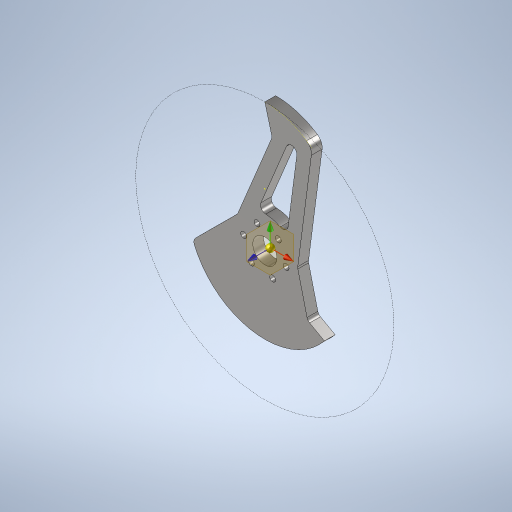
# Autodesk Inventor part: Blade
Saved by Autodesk Inventor 2023.4 (Build 274418000, 418)
## iProperties
Created: 2023-11-12
Part Number: Blade
Material: Steel, Alloy
Document SubType Name: Modeling
Designer: Nathan Cai
Density: 7.73 g/cm^3
Appearance: Semi-Polished
Mass: 199.265 g
Surface Area: 116.36 cm^2
Volume: 25.7782 cm^3
Author: Nathan Cai
Autodesk Inventor part; units mm, degrees
ref_plane "YZ Plane" through (0, 0, 0) normal (1, 0, 0) x (0, 1, 0)
ref_plane "XZ Plane" through (0, 0, 0) normal (0, 1, 0) x (-1, 0, 0)
ref_plane "XY Plane" through (0, 0, 0) normal (0, 0, 1) x (1, 0, 0)
sketch "Sketch1" plane through (0, 0, 0) normal (0, 0, 1) x (1, 0, 0)
  circle A0 centre (0, 0) radius 76.2 construction
  circle A1 centre (0, 0) radius 7.1437
  circle A2 centre (0, 0) radius 12.7 construction
  circle A3 centre (0, 0) radius 19.05
  line L0 (0, 76.2) -> (0, 0) construction
  line L1 (0, 76.2) -> (4.2947, 60.1719)
  line L2 (4.2947, 60.1719) -> (-17.6011, 7.2873)
  circle A4 centre (0, 0) radius 60.325 construction
  arc A5 (27.9352, 66.3249) -> (0, 76.2) centre (0, 31.75) ccw
  line L3 (27.9352, 66.3249) -> (18.8874, -2.4836)
  circle A6 centre (0, 0) radius 45.2437 construction
  line L4 (35.161, -28.4728) -> (0, 0) construction
  line L5 (35.161, -28.4728) -> (25.2413, -22.9743)
  line L6 (25.2413, -22.9743) -> (18.5029, 4.5327)
  circle A7 centre (0, 0) radius 34.1313 construction
  arc A8 (-42.5152, -15.4743) -> (35.161, -28.4728) centre (0, 0) ccw
  line L7 (-42.5152, -15.4743) -> (-13.4471, 13.4936)
  line L8 (-42.5152, -15.4743) -> (0, 0) construction
  line L9 (-4.3483, 18.5471) -> (12.7964, 59.9565)
  line L10 (13.0349, 13.8922) -> (18.8778, 58.328)
  arc A9 (18.8778, 58.328) -> (12.7964, 59.9565) centre (15.7299, 58.7419) ccw
  line L11 (-10.5541, 7.064) -> (0, 0) construction
  line L12 (0, 0) -> (-4.5937, 11.8401) construction
  circle A10 centre (-4.5937, 11.8401) radius 1.7526
  circle A11 centre (-12.5507, 1.9418) radius 1.7526
  circle A12 centre (-7.957, -9.8983) radius 1.7526
  circle A13 centre (4.5937, -11.8401) radius 1.7526
  circle A14 centre (12.5507, -1.9418) radius 1.7526
  circle A15 centre (7.957, 9.8983) radius 1.7526
  point P0 (19.3535, 1.0607)
  point P1 (-15.8759, 11.4541)
  point P2 (-16.1444, 10.8057)
  dimension "d0" = 152.4
  dimension "d14" = 15.875
  dimension "d17" = 68.2625
  dimension "d1" = 14.2875
  dimension "d2" = 25.4
  dimension "d8" = 38.1
  dimension "d9" = 15
  dimension "d11" = 44.45
  dimension "d12" = 15
  dimension "d15" = 90.4875
  dimension "d16" = 10
  dimension "d18" = 51
  dimension "d19" = 121
  dimension "d28" = 7.9375
  dimension "d29" = 7.9375
  dimension "d30" = 3.175
  dimension "d31" = 35
  dimension "d32" = 3.5052
  dimension "d35" = 360
  constraints: 26 end point, 16 point on circle, 13 centre point, 8 coincident, 6 tangent, 3 point on line, 2 concentric, 2 parallel, 1 vertical, 1 vertical alignment, 22 other
  measures "d1" diameter of A1
  measures "d2" diameter of A2
  measures "d8" diameter of A3
  measures "d9" angle of L0 L1
  measures "d11" radius of A5
  measures "d12" angle of L2 L3
  measures "d15" diameter of A6
  measures "d16" angle of L4 L5
  measures "d18" angle of L0 L4
  measures "d19" angle of L4 L8
  measures "d28" distance between parallel lines of L3 L10
  measures "d29" distance between parallel lines of L2 L9
  measures "d30" radius of A9
  measures "d31" angle of L11 L12
  measures "d32" diameter of A10
extrude "Extrusion1" add sketch "Sketch1" along normal blind 6.35 contours A3 | A3 L6 L3 | A3 L10 A9 L9 L7 L2 L1 A5 L3 L6 | L3 L6 L5 A8 L7 L2 A3 | L2 L7 A3
fillet "Fillet1" radius 3.175 6 edges at (19.3535, 1.0607, 3.175) (25.2413, -22.9743, 3.175) (4.2947, 60.1719, 3.175) (-4.3483, 18.5471, 3.175) (13.0349, 13.8922, 3.175) (-16.1444, 10.8057, 3.175)
fillet "Fillet3" radius 3.175 1 edges at (-42.5152, -15.4743, 3.175)
sketch "Sketch2" plane through (0, 0, 6.35) normal (0, 0, 1) x (1, 0, 0)
  arc A0 (27.9352, 66.3249) -> (0, 76.2) centre (0, 31.75) ccw construction
  circle A1 centre (0, 0) radius 76.2 construction
  constraints: 1 coincident, 1 vertical alignment, 2 other
fillet "Fillet4" radius 6.35 1 edges at (27.9352, 66.3249, 3.175)
equation "\"d29\" = d28"
body "Solid1"
